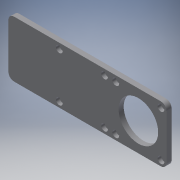
# Autodesk Inventor part: 30_Smartphone_Holder
Saved by Autodesk Inventor 2019 (Build 230136000, 136)
## iProperties
Created: 2019-07-16
Part Number: 30_Smartphone_Holder
Material: Generic
Document SubType Name: Modeling
Designer: marsikovabarbora
Density: 1 g/cm^3
Appearance: Default
Author: marsikovabarbora
Autodesk Inventor part; units mm, degrees
ref_plane "YZ Plane" through (0, 0, 0) normal (1, 0, 0) x (0, 1, 0)
ref_plane "XZ Plane" through (0, 0, 0) normal (0, 1, 0) x (-1, 0, 0)
ref_plane "XY Plane" through (0, 0, 0) normal (0, 0, 1) x (1, 0, 0)
sketch "Sketch1" plane through (0, 0, 0) normal (0, 0, 1) x (1, 0, 0)
  line L0 (-16.3829, -30.3318) -> (-62.1829, -30.3318)
  line L1 (-64.1829, -80.1318) -> (-14.3829, -80.1318) construction
  line L2 (35.6171, -80.1318) -> (-104.3829, -80.1318)
  line L3 (-104.3829, -80.1318) -> (-104.3829, -30.3318)
  line L4 (-104.3829, -30.3318) -> (35.6171, -30.3318)
  line L5 (35.6171, -30.3318) -> (35.6171, -80.1318)
  line L6 (-14.3829, -78.1318) -> (-14.3829, -32.3318)
  circle A0 centre (-19.2829, -75.2318) radius 1.4
  circle A1 centre (-59.2829, -75.2318) radius 1.4
  circle A2 centre (-19.2829, -35.2318) radius 1.4
  circle A3 centre (-59.2829, -35.2318) radius 1.4
extrude "Extrusion1" add sketch "Sketch1" along normal blind 4.5
sketch "Sketch4" plane through (0, 0, 4.5) normal (0, 0, 1) x (1, 0, 0)
  circle A0 centre (10.7171, -55.2318) radius 16.9 construction
  circle A1 centre (-9.2829, -35.2318) radius 1.45 projected
  circle A2 centre (30.7171, -35.2318) radius 1.45 projected
  arc A3 (-9.2829, -73.8318) -> (-9.2829, -76.6318) centre (-9.2829, -75.2318) ccw projected
  arc A4 (-9.2829, -73.8318) -> (-9.2829, -76.6318) centre (-9.2829, -75.2318) ccw projected
  arc A5 (30.7171, -76.6318) -> (30.7171, -73.8318) centre (30.7171, -75.2318) ccw projected
  circle A6 centre (30.7171, -75.2318) radius 1.4
  circle A7 centre (30.7171, -35.2318) radius 1.4
  circle A8 centre (-9.2829, -75.2318) radius 1.4
  circle A9 centre (-9.2829, -35.2318) radius 1.4
  circle A10 centre (10.7171, -55.2318) radius 17.5
  point P0 (0, 0)
  dimension "d44" = 2.8
  dimension "d45" = 2.8
  dimension "d46" = 2.8
  dimension "d47" = 2.8
  dimension "d48" = 35
  constraints: 5 centre point, 5 coincident
  measures "d44" diameter of A6
  measures "d45" diameter of A7
  measures "d46" diameter of A8
  measures "d47" diameter of A9
  measures "d48" diameter of A10
extrude "Extrusion3" cut sketch "Sketch4" against normal through all contours A8 A3 | A6 A5 | A7 | A9 | A10
sketch "Sketch3" plane through (0, 0, 4.5) normal (0, 0, 1) x (1, 0, 0)
  circle A0 centre (-9.2829, -35.2318) radius 1.4 projected
  circle A1 centre (-9.2829, -75.2318) radius 1.4 projected
  circle A2 centre (30.7171, -75.2318) radius 1.4 projected
  circle A3 centre (10.7171, -55.2318) radius 17.5 projected
  circle A4 centre (30.7171, -35.2318) radius 1.4 projected
  circle A5 centre (-59.2829, -35.2318) radius 1.4 projected
  circle A6 centre (-19.2829, -35.2318) radius 1.4 projected
  circle A7 centre (-59.2829, -75.2318) radius 1.4 projected
  circle A8 centre (-19.2829, -75.2318) radius 1.4 projected
  line L0 (-104.3829, -80.1318) -> (35.6171, -80.1318) projected
  line L1 (35.6171, -80.1318) -> (35.6171, -30.3318) projected
  line L2 (35.6171, -30.3318) -> (-104.3829, -30.3318) projected
  line L3 (-104.3829, -30.3318) -> (-104.3829, -80.1318) projected
  circle A9 centre (30.7171, -75.2318) radius 3
  circle A10 centre (-9.2829, -75.2318) radius 3
  circle A11 centre (-19.2829, -75.2318) radius 3
  circle A12 centre (-59.2829, -75.2318) radius 3
  circle A13 centre (30.7171, -35.2318) radius 3
  circle A14 centre (-9.2829, -35.2318) radius 3
  circle A15 centre (-19.2829, -35.2318) radius 3
  circle A16 centre (-59.2829, -35.2318) radius 3
  dimension "d51" = 1.6
  dimension "d52" = 1.6
  dimension "d53" = 1.6
  dimension "d54" = 1.6
  dimension "d55" = 1.6
  dimension "d56" = 1.6
  dimension "d57" = 1.6
  dimension "d58" = 1.6
  constraints: 8 centre point
  measures "d51" radial gap between concentric circles of A2 A9
  measures "d52" radial gap between concentric circles of A1 A10
  measures "d53" radial gap between concentric circles of A8 A11
  measures "d54" radial gap between concentric circles of A7 A12
  measures "d55" radial gap between concentric circles of A4 A13
  measures "d56" radial gap between concentric circles of A0 A14
  measures "d57" radial gap between concentric circles of A6 A15
  measures "d58" radial gap between concentric circles of A5 A16
extrude "Extrusion2" cut sketch "Sketch3" against normal blind 3.2 contours A9 | A10 | A11 | A12 | A13 | A14 | A15 | A16
fillet "Fillet1" radius 5 4 edges at (35.6171, -30.3318, 2.25) (-104.3829, -30.3318, 2.25) (-104.3829, -80.1318, 2.25) (35.6171, -80.1318, 2.25)
equation "\"d44\" = d40"
equation "\"d45\" = d40"
equation "\"d46\" = d40"
equation "\"d47\" = d40"
equation "\"d52\" = d51"
equation "\"d53\" = d51"
equation "\"d54\" = d51"
equation "\"d55\" = d51"
equation "\"d56\" = d51"
equation "\"d57\" = d51"
equation "\"d58\" = d51"
equation "\"d41\" = d40"
equation "\"d42\" = d40"
equation "\"d43\" = d40"
equation "\"d40\" = 2.8"
body "Solid1"
